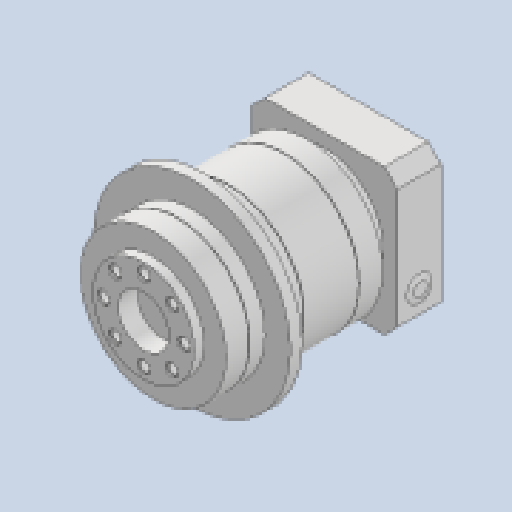
# Autodesk Inventor part: Gearbox
Saved by Autodesk Inventor 2025.2 (Build 292293000, 293)
## iProperties
Created: 2025-02-09
Part Number: Gearbox
Material: Generic
Document SubType Name: Modeling
Designer: LattePanda
Density: 1 g/cm^3
Appearance: Default
Author: LattePanda
Autodesk Inventor part; units mm, degrees
ref_plane "YZ Plane" through (0, 0, 0) normal (1, 0, 0) x (0, 1, 0)
ref_plane "XZ Plane" through (0, 0, 0) normal (0, 1, 0) x (-1, 0, 0)
ref_plane "XY Plane" through (0, 0, 0) normal (0, 0, 1) x (1, 0, 0)
sketch "Sketch1" plane through (0, 0, 0) normal (0, 0, 1) x (1, 0, 0)
  line L0 (-45, -45) -> (45, -45)
  line L1 (45, -45) -> (45, 45)
  line L2 (45, 45) -> (-45, 45)
  line L3 (-45, 45) -> (-45, -45)
  line L4 (-45, -45) -> (45, 45) construction
  line L5 (45, -45) -> (-45, 45) construction
  point P0 (0, 0)
  dimension "d0" = 90
  constraints: 12 end point, 2 midpoint, 2 parallel, 2 perpendicular, 1 horizontal
  measures "d0" distance of L1.end L2.end
extrude "Extrusion1" add sketch "Sketch1" along normal blind 27
chamfer "Chamfer1" distance 8 angle 45 4 edges at (45, 45, 13.5) (45, -45, 13.5) (-45, -45, 13.5) (-45, 45, 13.5)
sketch "Sketch2" plane through (0, 0, 27) normal (0, 0, 1) x (1, 0, 0)
  circle A0 centre (0, 0) radius 36.5
  dimension "d6" = 73
  constraints: 1 centre point, 1 coincident
  measures "d6" diameter of A0
extrude "Extrusion2" add sketch "Sketch2" along normal blind 11
sketch "Sketch3" plane through (0, 0, 38) normal (0, 0, 1) x (1, 0, 0)
  circle A0 centre (0, 0) radius 47
  dimension "d11" = 94
  constraints: 1 centre point, 1 coincident
  measures "d11" diameter of A0
extrude "Extrusion3" add sketch "Sketch3" along normal blind 15
chamfer "Chamfer2" distance 0.5 angle 45 1 edges at (-47, 0, 53)
sketch "Sketch4" plane through (0, 0, 53) normal (0, 0, 1) x (1, 0, 0)
  circle A0 centre (0, 0) radius 47 projected
extrude "Extrusion4" add sketch "Sketch4" along normal blind 34.25
chamfer "Chamfer3" distance 0.5 angle 45 1 edges at (-47, 0, 87.25)
sketch "Sketch5" plane through (0, 0, 87.25) normal (0, 0, 1) x (1, 0, 0)
  circle A0 centre (0, 0) radius 47 projected
extrude "Extrusion5" add sketch "Sketch5" along normal blind 15
sketch "Sketch6" plane through (0, 0, 102.25) normal (0, 0, 1) x (1, 0, 0)
  circle A0 centre (0, 0) radius 61
  circle A1 centre (0, 0) radius 47 projected
  dimension "d22" = 14
  constraints: 1 centre point, 1 coincident
  measures "d22" radial gap between concentric circles of A0 A1
extrude "Extrusion6" add sketch "Sketch6" along normal blind 7 contours A0 | A1
sketch "Sketch7" plane through (0, 0, 109.25) normal (0, 0, 1) x (1, 0, 0)
  circle A0 centre (0, 0) radius 45
  dimension "d25" = 90
  constraints: 1 centre point, 1 coincident
  measures "d25" diameter of A0
extrude "Extrusion7" add sketch "Sketch7" along normal blind 9.5
chamfer "Chamfer4" distance 0.5 angle 45 1 edges at (-45, 0, 118.75)
sketch "Sketch8" plane through (0, 0, 118.75) normal (0, 0, 1) x (1, 0, 0)
  circle A0 centre (0, 0) radius 45 projected
extrude "Extrusion8" add sketch "Sketch8" along normal blind 14.5
sketch "Sketch9" plane through (0, 0, 133.25) normal (0, 0, 1) x (1, 0, 0)
  circle A0 centre (0, 0) radius 31.5
  circle A1 centre (0, 0) radius 47 projected
  circle A2 centre (0, 0) radius 15.65
  dimension "d33" = 63
  dimension "d34" = 31.3
  constraints: 2 centre point, 2 coincident
  measures "d33" diameter of A0
  measures "d34" diameter of A2
extrude "Extrusion9" add sketch "Sketch9" along normal blind 6 contours A0
sketch "Sketch10" plane through (0, 0, 133.25) normal (0, 0, 1) x (1, 0, 0)
  circle A0 centre (0, 0) radius 15.65 projected
extrude "Extrusion10" cut sketch "Sketch10" against normal blind 6
sketch "Sketch11" plane through (0, 0, 139.25) normal (0, 0, 1) x (1, 0, 0)
  circle A0 centre (0, 0) radius 31.5 projected
  circle A1 centre (0, 0) radius 46.5 projected
  circle A2 centre (0, 0) radius 27.9 construction
  circle A3 centre (0, -24.9) radius 3
  line L0 (0, -85.4) -> (0, 85.4) construction
  circle A4 centre (0, 0) radius 24.9 construction
  circle A5 centre (17.607, -17.607) radius 3
  circle A6 centre (24.9, 0) radius 3
  circle A7 centre (17.607, 17.607) radius 3
  circle A8 centre (0, 24.9) radius 3
  circle A9 centre (-17.607, 17.607) radius 3
  circle A10 centre (-24.9, 0) radius 3
  circle A11 centre (-17.607, -17.607) radius 3
  circle A12 centre (-17.607, -17.607) radius 4
  circle A13 centre (0, -24.9) radius 4
  circle A14 centre (17.607, -17.607) radius 4
  circle A15 centre (24.9, 0) radius 4
  circle A16 centre (17.607, 17.607) radius 4
  circle A17 centre (-24.9, 0) radius 4
  circle A18 centre (-17.607, 17.607) radius 4
  circle A19 centre (0, 24.9) radius 4
  dimension "d39" = 3.6
  dimension "d40" = 6
  dimension "d43" = 360
  dimension "d47" = 8
  dimension "d48" = 8
  dimension "d49" = 8
  dimension "d50" = 8
  dimension "d51" = 8
  dimension "d52" = 8
  dimension "d53" = 8
  dimension "d54" = 8
  constraints: 17 centre point, 10 coincident, 1 point on line, 1 tangent, 1 vertical alignment, 19 other
  measures "d39" radial gap between concentric circles of A0 A2
  measures "d40" diameter of A3
  measures "d47" diameter of A12
  measures "d48" diameter of A13
  measures "d49" diameter of A14
  measures "d50" diameter of A15
  measures "d51" diameter of A16
  measures "d52" diameter of A17
  measures "d53" diameter of A18
  measures "d54" diameter of A19
extrude "Extrusion11" cut sketch "Sketch11" against normal blind 10 contours A3 | A5 | A6 | A7 | A8 | A9 | A10 | A11
extrude "Extrusion12" cut sketch "Sketch11" against normal blind 1 contours A3 | A5 | A6 | A7 | A8 | A9 | A10 | A11 | A12 | A13 | A14 | A15 | A16 | A17 | A18 | A19
sketch "Sketch12" plane through (45, -37, 0) normal (1, 0, 0) x (0, 0, -1)
  line L0 (-27, -8) -> (0, -8) projected
  line L1 (-13.5, -8) -> (-13.5, 14) construction
  circle A0 centre (-13.5, 14) radius 8
  point P0 (0, 37)
  dimension "d57" = 22
  dimension "d58" = 16
  constraints: 2 end point, 1 centre point, 1 coincident, 1 midpoint, 1 vertical
  measures "d57" distance of L1.start L1.end
  measures "d58" diameter of A0
extrude "Extrusion13" add sketch "Sketch12" along normal blind 1
fillet "Fillet1" radius 8 1 edges at (46, -23, 21.5)
mirror "Mirror1" about plane through (0, 0, 0) normal (1, 0, 0) of "Extrusion13", "Fillet1"
sketch "Sketch14" plane through (0, 0, 0) normal (0, 0, -1) x (-1, 0, 0)
  circle A0 centre (34.7985, -34.7985) radius 2.8 projected
  circle A1 centre (-34.7985, -34.7985) radius 2.8 projected
  circle A2 centre (-34.7985, 34.7985) radius 2.8 projected
  circle A3 centre (34.7985, 34.7985) radius 2.8 projected
  point P0 (0, 0)
hole "Hole1" at (-34.7985, -34.7985, 0) at (34.7985, -34.7985, 0) at (34.7985, 34.7985, 0) at (-34.7985, 34.7985, 0) direction (0, 0, 1) diameter 6 depth 10 tip angle 118
body "Solid1"
